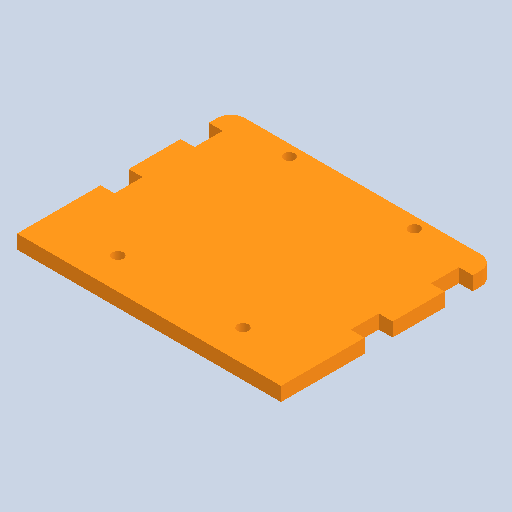
# Autodesk Inventor part: Top Base
Saved by Autodesk Inventor 2022 (Build 260153000, 153)
## iProperties
Created: 2021-07-09
Part Number: Top Base
Material: Glass
Document SubType Name: Modeling
Designer: benka
Density: 2.18 g/cm^3
Appearance: Orange
Author: benka
Autodesk Inventor part; units mm, degrees
ref_plane "YZ Plane" through (0, 0, 0) normal (1, 0, 0) x (0, 1, 0)
ref_plane "XZ Plane" through (0, 0, 0) normal (0, 1, 0) x (-1, 0, 0)
ref_plane "XY Plane" through (0, 0, 0) normal (0, 0, 1) x (1, 0, 0)
sketch "Sketch1" plane through (47.5, 0, 39.0178) normal (0, 1, 0) x (-1, 0, 0)
  line L0 (5, -58.8965) -> (0, -58.8965)
  line L1 (5, -69) -> (5, -58.8965)
  line L2 (5, -69) -> (0, -69)
  line L3 (0, -69) -> (0, -72)
  arc A0 (0, -72) -> (5, -77) centre (5, -72) ccw
  line L4 (5, -77) -> (90, -77)
  arc A1 (90, -77) -> (95, -72) centre (90, -72) ccw
  circle A2 centre (25, -73) radius 2
  circle A3 centre (70, -73) radius 2
  line L5 (0, 0) -> (95, 0)
  line L6 (0, -30.0747) -> (0, 0)
  line L7 (95, -40.1783) -> (95, -58.8965)
  line L8 (95, -30.0747) -> (95, 0)
  line L9 (0, -40.1783) -> (0, -58.8965)
  line L10 (90, -58.8965) -> (90, -69)
  line L11 (90, -58.8965) -> (95, -58.8965)
  line L12 (5, -30.0747) -> (0, -30.0747)
  line L13 (5, -40.1783) -> (5, -30.0747)
  line L14 (5, -40.1783) -> (0, -40.1783)
  line L15 (90, -40.1783) -> (95, -40.1783)
  line L16 (90, -30.0747) -> (90, -40.1783)
  line L17 (90, -30.0747) -> (95, -30.0747)
  line L18 (90, -69) -> (95, -69)
  line L19 (95, -72) -> (95, -69)
  circle A4 centre (25, -11.3502) radius 2
  circle A5 centre (70, -11.3502) radius 2
  point P0 (31.9525, -5.2817)
  dimension "d3" = 95
  constraints: 40 end point, 6 centre point, 4 point on circle
  measures "d3" distance between parallel lines of L9 L7
extrude "Top Base" add sketch "Sketch1" along normal blind 5
body "Solid1"
